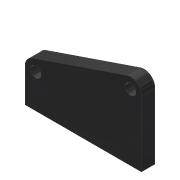
# Autodesk Inventor part: COXA_ROLL_COUPLER_BACK
Saved by Autodesk Inventor 2019.4 (Build 234330000, 330)
## iProperties
Created: 2019-10-21
Part Number: COXA_ROLL_COUPLER_BACK
Material: 一般
Document SubType Name: Modeling
Designer: y6tada
Density: 1 g/cm^3
Appearance: 濃い灰色
Author: y6tada
Autodesk Inventor part; units mm, degrees
ref_plane "YZ Plane" through (0, 0, 0) normal (1, 0, 0) x (0, 1, 0)
ref_plane "XZ Plane" through (0, 0, 0) normal (0, 1, 0) x (-1, 0, 0)
ref_plane "XY Plane" through (0, 0, 0) normal (0, 0, 1) x (1, 0, 0)
sketch "スケッチ1" plane through (0, 0, 0) normal (0, 0, 1) x (1, 0, 0)
  line L0 (0, 0) -> (35, 11.927) construction
  line L1 (33.7098, 15.7132) -> (-1.2902, 3.7862)
  line L2 (-4, 0) -> (-4, -12.5)
  line L3 (-4, -12.5) -> (39, -12.5)
  line L4 (39, -12.5) -> (39, 11.927)
  arc A0 (-1.2902, 3.7862) -> (-4, 0) centre (0, 0) ccw
  arc A1 (39, 11.927) -> (33.7098, 15.7132) centre (35, 11.927) ccw
  dimension "d0" = 35
  dimension "d1" = 11.927
  dimension "d2" = 4
  dimension "d12" = 12.5
  constraints: 10 end point, 4 coincident, 4 point on circle, 4 tangent, 2 centre point, 2 perpendicular, 1 equal radius, 1 horizontal
  measures "d0" horizontal distance of L0.end point (0, 0)
  measures "d1" vertical distance of point (0, 0) L0.end
  measures "d2" radius of A0
  measures "d12" distance from line of L3 point (0, 0)
extrude "押し出し1" add sketch "スケッチ1" along normal blind 5
hole "穴1" at (0, 0, 0) at (35, 11.927, 0) direction (0, 0, 1) diameter 4 end through all
